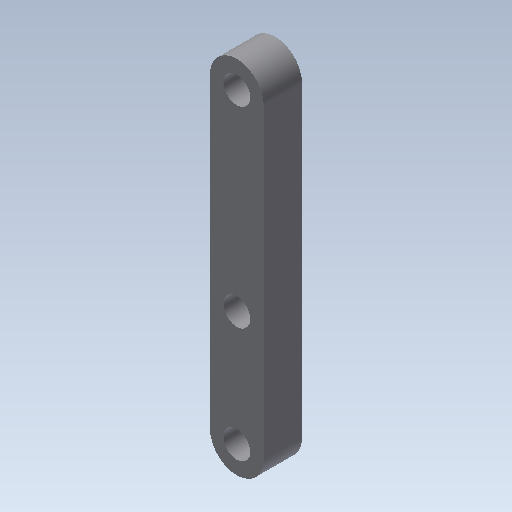
# Autodesk Inventor part: bar
Saved by Autodesk Inventor 2020.1 (Build 241239000, 239)
## iProperties
Created: 2016-10-14
Part Number: bar
Material: Generic
Document SubType Name: Modeling
Designer: Bardo91
Density: 1 g/cm^3
Appearance: Default
Author: Bardo91
Autodesk Inventor part; units mm, degrees
ref_plane "YZ Plane" through (0, 0, 0) normal (1, 0, 0) x (0, 1, 0)
ref_plane "XZ Plane" through (0, 0, 0) normal (0, 1, 0) x (-1, 0, 0)
ref_plane "XY Plane" through (0, 0, 0) normal (0, 0, 1) x (1, 0, 0)
sketch "Sketch1" plane through (0, 0, 0) normal (0, 0, 1) x (1, 0, 0)
  circle A0 centre (0, 0) radius 3.5
  line L0 (0, 0) -> (0, 40)
  circle A1 centre (0, 40) radius 3.5
  line L1 (3.5, 40) -> (3.5, 0)
  line L2 (-3.5, 40) -> (-3.5, 0)
  dimension "d0" = 7
  dimension "d1" = 40
  dimension "d2" = 7
  constraints: 6 end point, 4 point on circle, 2 centre point, 2 coincident, 2 tangent, 1 vertical
  measures "d0" diameter of A0
  measures "d1" distance of L0.start L0.end
  measures "d2" diameter of A1
extrude "Extrusion1" add sketch "Sketch1" along normal blind 5
sketch "Sketch2" plane through (0, 0, 5) normal (0, 0, 1) x (1, 0, 0)
  circle A0 centre (0, 0) radius 1.75
  arc A1 (3.5, 40) -> (-3.5, 40) centre (0, 40) ccw projected
  circle A2 centre (0, 40) radius 1.75
  dimension "d5" = 3.5
  dimension "d6" = 3.5
  constraints: 2 centre point, 2 coincident
  measures "d5" diameter of A0
  measures "d6" diameter of A2
extrude "Extrusion2" cut sketch "Sketch2" against normal blind 5
sketch "Sketch3" plane through (0, 0, 5) normal (0, 0, 1) x (1, 0, 0)
  line L0 (0, 0) -> (0, 15)
  circle A0 centre (0, 15) radius 1.75
  dimension "d9" = 15
  dimension "d10" = 3.5
  constraints: 2 end point, 1 centre point, 1 coincident, 1 vertical
  measures "d9" distance of L0.start L0.end
  measures "d10" diameter of A0
extrude "Extrusion3" cut sketch "Sketch3" against normal blind 10
body "Solid1"
